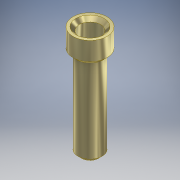
# Autodesk Inventor part: PinRecepticle-0.38-0.56mm
Saved by Autodesk Inventor 2018 (Build 220112000, 112)
## iProperties
Created: 2018-07-10
Part Number: PinRecepticle-0.38-0.56mm
Material: Copper
Document SubType Name: Modeling
Designer: Bradley
Density: 8.94 g/cm^3
Appearance: Gold - Metal
Author: Bradley
Autodesk Inventor part; units mm, degrees
ref_plane "YZ Plane" through (0, 0, 0) normal (1, 0, 0) x (0, 1, 0)
ref_plane "XZ Plane" through (0, 0, 0) normal (0, 1, 0) x (-1, 0, 0)
ref_plane "XY Plane" through (0, 0, 0) normal (0, 0, 1) x (1, 0, 0)
sketch "Sketch1" plane through (0, 0, 0) normal (0, 1, 0) x (-1, 0, 0)
  line L0 (0, -1.9685) -> (-0.3048, -1.9685)
  line L1 (-0.3048, -1.9685) -> (-0.4318, -1.8415)
  line L2 (-0.4318, -1.8415) -> (-0.4318, 1.1811)
  line L3 (-0.4318, 1.1811) -> (-0.4826, 1.1811)
  line L4 (-0.4826, 1.1811) -> (-0.6096, 1.3081)
  line L5 (-0.6096, 1.3081) -> (-0.6096, 1.9685)
  line L6 (-0.6096, 1.9685) -> (-0.508, 1.9685)
  line L7 (-0.508, 1.9685) -> (-0.381, 1.8415)
  line L8 (-0.381, 1.8415) -> (-0.381, -0.0635)
  line L9 (-0.381, -0.0635) -> (-0.2921, -0.1524)
  line L10 (-0.2921, -0.1524) -> (-0.2921, -1.5367)
  line L11 (-0.2921, -1.5367) -> (0, -1.7122)
  line L12 (0, -1.7122) -> (0, -1.9685)
  line L13 (0, -1.9685) -> (0, 1.9685) construction
  point P0 (0, 0)
  point P1 (0, 0)
  dimension "d0" = 1.2192
  dimension "d1" = 0.7874
  dimension "d2" = 2.032
  dimension "d3" = 3.937
  dimension "d4" = 3.5052
  dimension "d5" = 59
  dimension "d6" = 135
  dimension "d7" = 0.8636
  dimension "d8" = 0.5842
  dimension "d9" = 0.127
  dimension "d10" = 0.762
  dimension "d11" = 1.016
  constraints: 28 end point, 8 parallel, 3 perpendicular, 1 coincident, 1 horizontal, 1 midpoint, 1 point on line, 1 vertical
  measures "d0" diameter of L5 L13
  measures "d1" distance between parallel lines of L3 L6
  measures "d2" distance from line of L8.end L6
  measures "d3" distance between parallel lines of L0 L6
  measures "d4" distance from line of L10.end L6
  measures "d5" angle of L13 L11
  measures "d6" angle of L0 L1
  measures "d7" diameter of L2 L13
  measures "d8" diameter of L10 L13
  measures "d9" horizontal distance of L0.end L1.end
  measures "d10" diameter of L8 L13
  measures "d11" diameter of L6.end L13
revolve "Revolution1" add sketch "Sketch1" angle 360 about axis through (0, 0, -1.7122) along (0, 0, -1)
body "Solid1"
